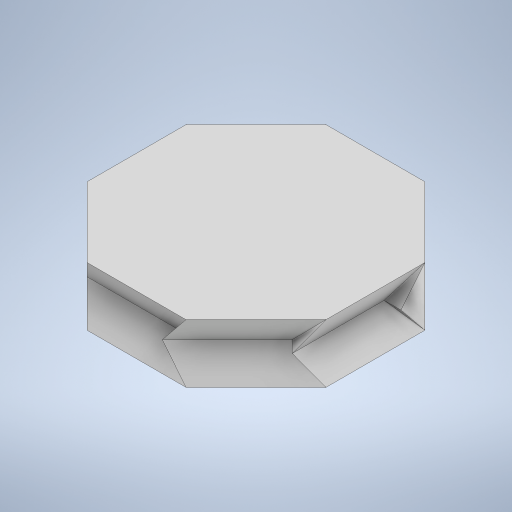
# Autodesk Inventor part: 팔각형 OV-PAM 층 한개
Saved by Autodesk Inventor 2024 (Build 280153000, 153)
## iProperties
Created: 2023-06-16
Part Number: 팔각형 OV-PAM 층 한개
Material: 일반
Document SubType Name: Modeling
Designer: jsw
Density: 1 g/cm^3
Appearance: 기본값
Author: jsw
Autodesk Inventor part; units mm, degrees
sketch "스케치1" plane through (0, 0, 0) normal (0, 1, 0) x (-1, 0, 0)
  line L0 (-31.9919, 13.2515) -> (-13.2515, 31.9919)
  line L1 (-13.2515, 31.9919) -> (13.2515, 31.9919)
  line L2 (13.2515, 31.9919) -> (31.9919, 13.2515)
  line L3 (31.9919, 13.2515) -> (31.9919, -13.2515)
  line L4 (31.9919, -13.2515) -> (13.2515, -31.9919)
  line L5 (13.2515, -31.9919) -> (-13.2515, -31.9919)
  line L6 (-13.2515, -31.9919) -> (-31.9919, -13.2515)
  line L7 (-31.9919, -13.2515) -> (-31.9919, 13.2515)
  line L8 (-13.5, 32.5919) -> (13.5, 32.5919)
  line L9 (13.5, 32.5919) -> (32.5919, 13.5)
  line L10 (32.5919, 13.5) -> (32.5919, -13.5)
  line L11 (32.5919, -13.5) -> (13.5, -32.5919)
  line L12 (13.5, -32.5919) -> (-13.5, -32.5919)
  line L13 (-13.5, -32.5919) -> (-32.5919, -13.5)
  line L14 (-32.5919, -13.5) -> (-32.5919, 13.5)
  line L15 (-32.5919, 13.5) -> (-13.5, 32.5919)
  point P0 (0, 0)
  point P1 (0, 0)
  point P2 (0, 0)
  dimension "d2" = 0.6
  dimension "d62" = 27
  constraints: 32 end point, 2 coincident, 2 horizontal, 34 other
  measures "d2" distance between parallel lines of L10 L3
  measures "d62" distance of L11.end L12.end
extrude "돌출2" add sketch "스케치1" along normal blind 8 contours L0 L1 L2 L3 L4 L5 L6 L7 | L8 L9 L10 L11 L12 L13 L14 L15
ref_plane "작업 평면2" through (32.5919, 0, 13.5) normal (-0.8660254, -0.5, 0) x (0, 0, -1)
sketch "스케치4" plane through (13.5, 0, 32.5919) normal (0.7071068, 0, 0.7071068) x (0.7071068, 0, -0.7071068)
  line L0 (0, 0) -> (0, 8) projected
  line L1 (27, 0) -> (27, 8) projected
  line L2 (0, 0) -> (27, 0)
  line L3 (27, 0) -> (27, 8)
  line L4 (27, 8) -> (0, 8)
  line L5 (0, 8) -> (0, 0)
  line L6 (27, 0) -> (20.5, 8)
  line L7 (27, 0) -> (0, 0) projected
  line L8 (0, 0) -> (-21.9798, 8)
  line L9 (27, 8) -> (0, 8) projected
  line L10 (0, 8) -> (-19.0919, 8) projected
  line L11 (0, 8) -> (-21.9798, 8)
  line L12 (0, 8) -> (27, 8) projected
  point P0 (13.5, 0)
  point P1 (8.7224, 21)
  point P2 (13.5, 8)
  point P3 (13.5, 8)
  point P4 (13.5, 8)
  dimension "d44" = 160
  dimension "d61" = 7
  constraints: 14 end point, 3 midpoint, 2 parallel, 2 point on line, 1 collinear, 1 horizontal, 1 perpendicular
  measures "d44" angle of L8 L2
  measures "d61" distance of point (13.5, 8) L6.end
ref_plane "작업 평면7" through (13.5, 0, 32.5919) normal (-0.6123724, -0.5, -0.6123724) x (0.7071068, 0, -0.7071068)
extrude "돌출10" cut sketch "스케치4" against normal up to surface contours L8 L11 L10 L0 | L0 L4 L6 L2 surface through (13.5, 0, 32.5919) normal (-0.6123724, -0.5, -0.6123724)
pattern_circular "원형 패턴3" count 8 over 360 about axis through (0, -10, 0) along (0, 1, 0) of "돌출10"
mirror "미러8" about plane through (0, 8, 0) normal (0, 1, 0) of "돌출10", "원형 패턴3", "돌출2"
ref_plane "작업 평면8" through (0, 8, 0) normal (0, -1, 0) x (1, 0, 0)
